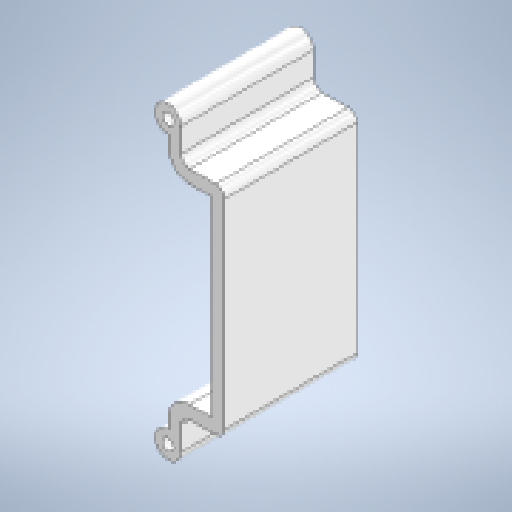
# Autodesk Inventor part: mune_1
Saved by Autodesk Inventor 2025.1 (Build 291241000, 241)
## iProperties
Created: 2024-09-03
Part Number: mune_1
Material: ABS プラスチック
Document SubType Name: Modeling
Designer: right
Density: 1.06 g/cm^3
Appearance: 滑らか - 黒
Mass: 8.92511 g
Surface Area: 66.7912 cm^2
Volume: 8.41992 cm^3
Author: right
Autodesk Inventor part; units mm, degrees
ref_plane "YZ Plane" through (0, 0, 0) normal (1, 0, 0) x (0, 1, 0)
ref_plane "XZ Plane" through (0, 0, 0) normal (0, 1, 0) x (-1, 0, 0)
ref_plane "XY Plane" through (0, 0, 0) normal (0, 0, 1) x (1, 0, 0)
sketch "スケッチ1" plane through (0, 0, 0) normal (0, 0, 1) x (1, 0, 0)
  circle A0 centre (-7.5, 32.5) radius 1.6 projected
  circle A1 centre (7.5, -32.5) radius 1.6 projected
  circle A2 centre (7.5, 32.5) radius 1.6 projected
  circle A3 centre (-7.5, -32.5) radius 1.6 projected
  circle A4 centre (15.5, 0) radius 1.1 projected
  circle A5 centre (10.5, -5) radius 1.1 projected
  circle A6 centre (5.5, 0) radius 1.1 projected
  circle A7 centre (10.5, 5) radius 1.1 projected
  arc A8 (-10.5, -38) -> (-8.5, -40) centre (-8.5, -38) ccw projected
  line L0 (-8.5, -40) -> (8.5, -40) projected
  arc A9 (8.5, -40) -> (10.5, -38) centre (8.5, -38) ccw projected
  line L1 (10.5, -38) -> (10.5, -27) projected
  arc A10 (12.5, -25) -> (10.5, -27) centre (12.5, -27) ccw projected
  line L2 (12.5, -25) -> (18.5, -25) projected
  arc A11 (18.5, -25) -> (20.5, -23) centre (18.5, -23) ccw projected
  line L3 (20.5, -23) -> (20.5, 23) projected
  arc A12 (20.5, 23) -> (18.5, 25) centre (18.5, 23) ccw projected
  line L4 (18.5, 25) -> (12.5, 25) projected
  arc A13 (10.5, 27) -> (12.5, 25) centre (12.5, 27) ccw projected
  line L5 (10.5, 27) -> (10.5, 38) projected
  arc A14 (10.5, 38) -> (8.5, 40) centre (8.5, 38) ccw projected
  line L6 (8.5, 40) -> (-8.5, 40) projected
  arc A15 (-8.5, 40) -> (-10.5, 38) centre (-8.5, 38) ccw projected
  line L7 (-10.5, 38) -> (-10.5, 27) projected
  arc A16 (-12.5, 25) -> (-10.5, 27) centre (-12.5, 27) ccw projected
  line L8 (-12.5, 25) -> (-27.5, 25) projected
  arc A17 (-27.5, 25) -> (-29.5, 23) centre (-27.5, 23) ccw projected
  line L9 (-29.5, 23) -> (-29.5, -23) projected
  arc A18 (-29.5, -23) -> (-27.5, -25) centre (-27.5, -23) ccw projected
  line L10 (-27.5, -25) -> (-12.5, -25) projected
  arc A19 (-10.5, -27) -> (-12.5, -25) centre (-12.5, -27) ccw projected
  line L11 (-10.5, -27) -> (-10.5, -38) projected
  circle A20 centre (-8, 38) radius 1.1 projected
  circle A21 centre (-8, -38) radius 1.1 projected
  circle A22 centre (8, -38) radius 1.1 projected
  circle A23 centre (8, 38) radius 1.1 projected
  circle A24 centre (7.5, -32.5) radius 3
  circle A25 centre (7.5, 32.5) radius 3
  line L12 (12.5, 22) -> (17.5, 22)
  line L13 (17.5, 22) -> (17.5, -22)
  line L14 (17.5, -22) -> (12.5, -22)
  arc A26 (12.5, -22) -> (7.5, -27) centre (12.5, -27) ccw
  line L15 (7.5, -27) -> (7.5, -37)
  line L16 (7.5, -37) -> (-7.5, -37)
  line L17 (-7.5, -37) -> (-7.5, -27)
  arc A27 (-7.5, -27) -> (-12.5, -22) centre (-12.5, -27) ccw
  line L18 (-12.5, -22) -> (-26.5, -22)
  line L19 (-26.5, -22) -> (-26.5, 22)
  line L20 (-26.5, 22) -> (-12.5, 22)
  arc A28 (-12.5, 22) -> (-7.5, 27) centre (-12.5, 27) ccw
  line L21 (-7.5, 27) -> (-7.5, 37)
  line L22 (-7.5, 37) -> (7.5, 37)
  line L23 (7.5, 37) -> (7.5, 27)
  arc A29 (7.5, 27) -> (12.5, 22) centre (12.5, 27) ccw
  circle A30 centre (7.5, -32.5) radius 1.3
  circle A31 centre (7.5, 32.5) radius 1.3
  point P0 (0, 0)
  point P1 (7.5, -29.5)
  point P2 (10.5, -32.5)
  point P3 (10.5, 32.5)
  point P4 (7.5, 29.5)
  point P5 (17.5, 0.4583)
  point P6 (17.5, -0.4583)
  point P7 (7.5, -33.8)
  point P8 (7.5, -31.2)
  point P9 (7.5, -30.9)
  point P10 (7.5, -34.1)
  point P11 (7.5, 35.5)
  point P12 (7.5, -35.5)
  dimension "d0" = 6
  dimension "d1" = 6
  dimension "d2" = 3
  dimension "d5" = 2.6
  dimension "d6" = 2.6
  constraints: 24 end point, 8 centre point, 8 point on circle, 4 coincident, 15 other
  measures "d0" diameter of A24
  measures "d1" diameter of A25
  measures "d2" radial gap between concentric circles of A13 A29
  measures "d5" diameter of A30
  measures "d6" diameter of A31
ref_plane "作業平面1" through (-29.5, -40, 30.5) normal (0, 0, -1) x (0, 1, 0)
extrude "押し出し1" add sketch "スケッチ1" along normal up to surface (30.5 mm away) contours L23 A2 A25 | A25 L23 A2 | L5 A13 L4 A12 L3 A11 L2 A10 L1 A24 L15 A26 L14 L13 L12 A29 L23 A25 | L23 A31 A2 | A2 L23 A31 | L15 A1 A24 | A24 L15 A1 | L15 A30 A1 | A1 L15 A30
